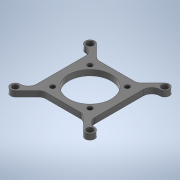
# Autodesk Inventor part: Fan_support_stand
Saved by Autodesk Inventor 2020.4 (Build 244396000, 396)
## iProperties
Created: 2022-05-23
Part Number: Fan_support_stand
Material: 一般
Document SubType Name: Modeling
Designer: Masato Kubotera
Density: 1 g/cm^3
Appearance: 滑らか - 黒
Author: Masato Kubotera
Autodesk Inventor part; units mm, degrees
ref_plane "YZ Plane" through (0, 0, 0) normal (1, 0, 0) x (0, 1, 0)
ref_plane "XZ Plane" through (0, 0, 0) normal (0, 1, 0) x (-1, 0, 0)
ref_plane "XY Plane" through (0, 0, 0) normal (0, 0, 1) x (1, 0, 0)
sketch "スケッチ1" plane through (0, 0, 0) normal (0, 0, 1) x (1, 0, 0)
  line L0 (10, -10) -> (-10, -10) construction
  line L1 (-10, -10) -> (-10, 10) construction
  line L2 (-10, 10) -> (10, 10) construction
  line L3 (10, 10) -> (10, -10) construction
  line L4 (10, -10) -> (-10, 10) construction
  line L5 (-10, -10) -> (10, 10) construction
  line L6 (12.5, -12.5) -> (-12.5, -12.5) construction
  line L7 (-12.5, -12.5) -> (-12.5, 12.5) construction
  line L8 (-12.5, 12.5) -> (12.5, 12.5) construction
  line L9 (12.5, 12.5) -> (12.5, -12.5) construction
  line L10 (12.5, -12.5) -> (-12.5, 12.5) construction
  line L11 (-12.5, -12.5) -> (12.5, 12.5) construction
  circle A0 centre (10, 10) radius 1.25
  circle A1 centre (-10, 10) radius 1.25
  circle A2 centre (10, -10) radius 1.25
  circle A3 centre (-10, -10) radius 1.25
  circle A4 centre (20, 20) radius 1.75
  line L12 (20, -20) -> (-20, -20) construction
  line L13 (-20, -20) -> (-20, 20) construction
  line L14 (-20, 20) -> (20, 20) construction
  line L15 (20, 20) -> (20, -20) construction
  line L16 (20, -20) -> (-20, 20) construction
  line L17 (-20, -20) -> (20, 20) construction
  circle A5 centre (-20, 20) radius 1.6
  circle A6 centre (20, -20) radius 1.75
  circle A7 centre (-20, -20) radius 1.75
  arc A8 (21.7678, 18.2322) -> (17.5, 20) centre (20, 20) ccw
  line L18 (17.5, 20) -> (17.5, 20)
  line L19 (13, 15.5) -> (-13, 15.5)
  circle A9 centre (0, 0) radius 11.3921
  arc A10 (13, 15.5) -> (17.5, 20) centre (13, 20) ccw
  line L20 (21.7678, 18.2322) -> (15.5637, 12.0282)
  line L21 (14.3921, 9.1997) -> (14.3921, -9.1997)
  arc A11 (15.5637, 12.0282) -> (14.3921, 9.1997) centre (18.3921, 9.1997) ccw
  line L22 (20, 0) -> (-20, 0) construction
  line L23 (0, 20) -> (0, -20) construction
  arc A12 (17.5, -20) -> (21.7678, -18.2322) centre (20, -20) ccw
  line L24 (17.5, -20) -> (17.5, -20)
  line L25 (13, -15.5) -> (-13, -15.5)
  arc A13 (17.5, -20) -> (13, -15.5) centre (13, -20) ccw
  line L26 (21.7678, -18.2322) -> (15.5637, -12.0282)
  arc A14 (14.3921, -9.1997) -> (15.5637, -12.0282) centre (18.3921, -9.1997) ccw
  circle A15 centre (10, 10) radius 2.75 construction
  arc A16 (-17.5, 20) -> (-21.7678, 18.2322) centre (-20, 20) ccw
  arc A17 (-17.5, 20) -> (-13, 15.5) centre (-13, 20) ccw
  line L27 (-21.7678, 18.2322) -> (-15.5637, 12.0282)
  line L28 (-14.3921, 9.1997) -> (-14.3921, -9.1997)
  arc A18 (-14.3921, 9.1997) -> (-15.5637, 12.0282) centre (-18.3921, 9.1997) ccw
  arc A19 (-15.5637, -12.0282) -> (-14.3921, -9.1997) centre (-18.3921, -9.1997) ccw
  line L29 (-21.7678, -18.2322) -> (-15.5637, -12.0282)
  arc A20 (-21.7678, -18.2322) -> (-17.5, -20) centre (-20, -20) ccw
  line L30 (-17.5, -20) -> (-17.5, -20)
  arc A21 (-13, -15.5) -> (-17.5, -20) centre (-13, -20) ccw
  line L31 (-17.5, 20) -> (-17.5, 20)
  dimension "d0" = 20
  dimension "d1" = 20
  dimension "d2" = 25
  dimension "d3" = 25
  dimension "d4" = 2.5
  dimension "d5" = 2.5
  dimension "d6" = 2.5
  dimension "d7" = 2.5
  dimension "d8" = 3.5
  dimension "d9" = 40
  dimension "d10" = 40
  dimension "d11" = 3.2
  dimension "d12" = 3.5
  dimension "d13" = 3.5
  dimension "d14" = 2.5
  dimension "d18" = 4
  dimension "d19" = 3
  dimension "d20" = 45
  dimension "d21" = 5.5
  dimension "d22" = 3
  constraints: 64 end point, 28 symmetric about line, 24 point on circle, 22 centre point, 11 coincident, 10 midpoint, 6 parallel, 6 tangent, 4 perpendicular, 3 horizontal, 2 point on line, 2 vertical, 9 other
  measures "d0" distance of L1.end L2.end
  measures "d1" distance of L0.end L1.end
  measures "d2" distance of L7.end L8.end
  measures "d3" distance of L6.end L7.end
  measures "d4" diameter of A0
  measures "d5" diameter of A1
  measures "d6" diameter of A2
  measures "d7" diameter of A3
  measures "d8" diameter of A4
  measures "d9" distance of L13.end L14.end
  measures "d10" distance of L12.end L13.end
  measures "d11" diameter of A5
  measures "d12" diameter of A6
  measures "d13" diameter of A7
  measures "d14" radius of A8
  measures "d18" radius of A11
  measures "d19" distance edge to line of A9 L21
  measures "d20" angle of L15 L20
  measures "d21" diameter of A15
  measures "d22" distance between parallel lines of L19 L8
extrude "押し出し1" add sketch "スケッチ1" along normal blind 3
equation "\"d1\" = d0"
equation "\"d3\" = d2"
equation "\"d5\" = d4"
equation "\"d6\" = d4"
equation "\"d7\" = d4"
equation "\"d22\" = d19"
